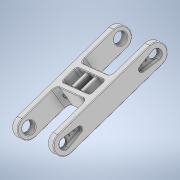
# Autodesk Inventor part: LegMiddle_Final_2
Saved by Autodesk Inventor 2020.3 (Build 243373000, 373)
## iProperties
Created: 2021-02-18
Part Number: LegMiddle_Final_2
Material: Generic
Document SubType Name: Modeling
Designer: sanyi
Density: 1 g/cm^3
Appearance: Default
Author: sanyi
Autodesk Inventor part; units mm, degrees
note: some values were not read from the file. Chosen so that the rebuilt part matches the saved one: direction of "Hole7"; direction of "Hole6".
ref_plane "YZ Plane" through (0, 0, 0) normal (1, 0, 0) x (0, 1, 0)
ref_plane "XZ Plane" through (0, 0, 0) normal (0, 1, 0) x (-1, 0, 0)
ref_plane "XY Plane" through (0, 0, 0) normal (0, 0, 1) x (1, 0, 0)
sketch "Sketch1" plane through (0, 0, 0) normal (0, 1, 0) x (-1, 0, 0)
  line L0 (0, 0) -> (0, 15.1754) construction
  line L1 (0, 0) -> (0, -18.4224) construction
  line L2 (0, 0) -> (12.9194, 0) construction
  line L3 (45, 17) -> (45, 23)
  line L4 (10, 17) -> (45, 17)
  line L5 (10, -17) -> (45, -17)
  line L6 (45, -17) -> (45, -23)
  line L7 (0, 0) -> (-12.9194, 0) construction
  line L8 (-45, 17) -> (-45, 23)
  line L9 (-10, 17) -> (-45, 17)
  line L10 (-10, -17) -> (-45, -17)
  line L11 (-45, -17) -> (-45, -23)
  line L12 (10, -17) -> (10, 17)
  line L13 (-10, -17) -> (-10, 17)
  line L14 (63, 0) -> (-63, 0) projected
  line L15 (-45, 23) -> (45, 23)
  line L16 (45, -23) -> (-45, -23)
  line L17 (-45, 34.0051) -> (-45, -29.7103) construction
  line L18 (45, 30.9627) -> (45, -32.2261) construction
  line L19 (0, -45.4724) -> (0, 47.2514) projected
  line L20 (45, 20) -> (-45, 20) construction
  dimension "d2" = 6
  dimension "d8" = 34
  dimension "d11" = 20
  dimension "d30" = 35
  dimension "d31" = 35
  constraints: 38 end point, 11 perpendicular, 6 point on line, 2 vertical, 6 other
  measures "d2" distance of L3.start L3.end
  measures "d8" distance of L4.start L5.start
  measures "d11" distance between parallel lines of L13 L12
  measures "d30" distance between parallel lines of L17 L13
  measures "d31" distance between parallel lines of L18 L12
extrude "Extrusion1" add sketch "Sketch1" along normal blind 15
sketch "Sketch2" plane through (0, 15, 0) normal (0, 1, 0) x (1, 0, 0)
  line L0 (-63, 0) -> (63, 0) projected
  line L1 (0, 32.2) -> (0, -32.2) projected
  line L2 (-6, -3) -> (6, -3)
  line L3 (6, -3) -> (6, 3)
  line L4 (6, 3) -> (-6, 3)
  line L5 (-6, 3) -> (-6, -3)
  line L6 (-6, -16) -> (6, -16)
  line L7 (6, -16) -> (6, -7)
  line L8 (6, -7) -> (-6, -7)
  line L9 (-6, -7) -> (-6, -16)
  line L10 (-6, 16) -> (6, 16)
  line L11 (6, 16) -> (6, 7)
  line L12 (6, 7) -> (-6, 7)
  line L13 (-6, 7) -> (-6, 16)
  line L14 (-6, -7) -> (-6, -3)
  line L15 (6, -7) -> (6, -3)
  line L16 (6, 3) -> (6, 7)
  line L17 (-6, 3) -> (-6, 7)
  line L18 (-10, -17) -> (-45, -17) projected
  point P0 (0, 0)
  dimension "d14" = 3
  dimension "d15" = 6
  dimension "d16" = 4
  dimension "d72" = 1
  constraints: 32 end point, 4 symmetric about line, 3 perpendicular, 2 collinear, 2 parallel, 1 horizontal, 1 vertical, 2 other
  measures "d14" distance between parallel lines of L4 L0
  measures "d15" distance between parallel lines of L3 L1
  measures "d16" distance between parallel lines of L2 L8
  measures "d72" distance between parallel lines of L18 L6
extrude "Extrusion2" cut sketch "Sketch2" against normal up to surface (15 mm away) contours L5 L4 L1 L0 | L0 L1 L2 L5 | L1 L4 L3 L0 | L0 L3 L2 L1 | L13 L10 L1 L12 | L8 L1 L6 L9 | L1 L10 L11 L12 | L8 L7 L6 L1
full round fillet "Fillet1" first side at (3.3333, 15, -21) centre faces at (-45, 5, -21) second side at (3.3333, 0, -21)
full round fillet "Fillet2" first side at (3.3333, 15, 21) centre faces at (45, 5, -19) second side at (3.3333, 0, 21)
full round fillet "Fillet3" first side at (3.3333, 15, 21) centre faces at (45, 5, 21) second side at (3.3333, 0, 21)
full round fillet "Fillet4" first side at (0.8334, 15, 21) centre faces at (-45, 5, 19) second side at (0.8334, 0, 21)
sketch "Sketch5" plane through (-37.5, 7.5, -23) normal (0, 0, -1) x (-1, 0, 0)
  arc A0 (0, -7.5) -> (0, 7.5) centre (0, 0) ccw projected
  arc A1 (-75, 7.5) -> (-75, -7.5) centre (-75, 0) ccw projected
  line L0 (-75, 0) -> (0, 0) construction
  circle A2 centre (0, 0) radius 3.6
  arc A3 (-12.3676, 1.8305) -> (-12.3676, -1.8305) centre (-12.1, 0) ccw
  line L1 (-0.5207, 3.5621) -> (-12.3676, 1.8305)
  line L2 (-12.3676, -1.8305) -> (-0.5207, -3.5621)
  circle A4 centre (-75, 0) radius 3.6
  arc A5 (-62.6324, -1.8305) -> (-62.6324, 1.8305) centre (-62.9, 0) ccw
  line L3 (-74.4793, 3.5621) -> (-62.6324, 1.8305)
  line L4 (-74.4793, -3.5621) -> (-62.6324, -1.8305)
  line L5 (-37.5, -7.5) -> (-37.5, 7.5)
  line L6 (-43.5, 7.5) -> (-31.5, 7.5) projected
  dimension "d53" = 3.7
  dimension "d54" = 12.1
  dimension "d76" = 12.1
  dimension "d89" = 7.2
  constraints: 12 end point, 8 point on circle, 8 tangent, 4 centre point, 2 coincident, 2 equal radius, 2 point on line, 1 horizontal, 1 midpoint
  measures "d53" diameter of A5
  measures "d54" distance of A5.centre L0.start
  measures "d76" distance of L0.end A3.centre
  measures "d89" diameter of A4
extrude "Extrusion4" cut sketch "Sketch5" against normal up to surface (6 mm away) contours A2 | A4
extrude "Extrusion5" cut sketch "Sketch5" against normal blind 3.5 contours A2 L2 A3 L1 | A4 L3 A5 L4
sketch "Sketch14" plane through (-37.5, 7.5, -19.5) normal (0, 0, -1) x (-1, 0, 0)
  arc A0 (-62.6324, -1.8305) -> (-62.6324, 1.8305) centre (-62.9, 0) ccw projected
  arc A1 (-12.3676, 1.8305) -> (-12.3676, -1.8305) centre (-12.1, 0) ccw projected
  line L0 (-62.9, 0) -> (-64.9, 0)
  line L1 (-12.1, 0) -> (-10.1, 0)
  line L2 (0, 7.5) -> (-75, 7.5) projected
  line L3 (0, -7.5) -> (-75, -7.5) projected
  line L4 (-37.5, 7.5) -> (-37.5, -7.5) construction
  line L5 (-75, 7.5) -> (-75, -7.5) construction
  line L6 (0, 7.5) -> (0, -7.5) construction
  line L7 (-75, 0) -> (0, 0) construction
  line L8 (-64.9, 0) -> (-66.9, 0)
  line L9 (-66.9, 0) -> (-68.9, 0)
  line L10 (-10.1, 0) -> (-8.1, 0)
  line L11 (-8.1, 0) -> (-6.1, 0)
  point P0 (-37.5, -7.5)
  point P1 (-12.1, 0)
  dimension "d121" = 2
  dimension "d122" = 2
  dimension "d123" = 2
  constraints: 20 end point, 8 coincident, 4 midpoint, 3 point on line, 3 symmetric about line, 2 vertical, 1 other
  measures "d121" distance of L0.start L0.end
  measures "d122" distance of L8.start L8.end
  measures "d123" distance of L8.end L9.end
hole "Hole7" at (27.4, 7.5, -19.5) at (31.4, 7.5, -19.5) at (-27.4, 7.5, -19.5) at (-31.4, 7.5, -19.5) direction (0, 0, 1) diameter 1 depth 2.5
extrude "Extrusion6" cut sketch "Sketch2" against normal blind 1 contours L17 L12 L1 L4 | L2 L1 L8 L14 | L1 L12 L16 L4 | L2 L15 L8 L1
sketch "Sketch6" plane through (0, 0, 0) normal (0, -1, 0) x (1, 0, 0)
  line L0 (6, 3) -> (6, 7) projected
  line L1 (6, 7) -> (-6, 7) projected
  line L2 (-6, 3) -> (6, 3) projected
  line L3 (-6, 7) -> (-6, 3) projected
  line L4 (6, -3) -> (-6, -3) projected
  line L5 (-6, -7) -> (6, -7) projected
  line L6 (-6, -3) -> (-6, -7) projected
  line L7 (6, -7) -> (6, -3) projected
  point P0 (0, 0)
extrude "Extrusion7" cut sketch "Sketch6" against normal blind 1
sketch "Sketch12" plane through (10, 0, 17) normal (1, 0, 0) x (0, 0, -1)
  line L0 (0, 0) -> (0, 15) projected
  line L1 (0, 7.5) -> (3, 7.5) construction
  point P0 (17, 0)
  dimension "d97" = 3
  constraints: 2 end point, 1 coincident, 1 horizontal, 1 midpoint
  measures "d97" distance of L1.start L1.end
hole "Hole5" at (10, 7.5, 14) direction (-1, 0, 0) diameter 3 end through all
fillet "Fillet13" radius 3.5 4 edges at (10, 7.5, 17) (-10, 7.5, 17) (-10, 7.5, -17) (10, 7.5, -17)
fillet "Fillet11" radius 2 4 edges at (-6, 7.5, -16) (6, 7.5, -16) (6, 7.5, 16) (-6, 7.5, 16)
fillet "Fillet9" radius 0.5 24 edges at (-6, 1, -5) (0, 1, -7) (0, 1, -3) (-6, 7.5, 3) (-6, 7.5, -7) (-6, 7.5, -3) (0, 14, -7) (0, 14, -3) (0, 1, 3) (0, 1, 7) (6, 1, -5) (6, 1, 5) (6, 7.5, -7) (6, 7.5, -3) (-6, 14, -5) (-6, 14, 5) (-6, 7.5, 7) (0, 14, 7) (0, 14, 3) (6, 14, 5) (6, 7.5, 3) (6, 7.5, 7) (-6, 1, 5) (6, 14, -5)
fillet "Fillet15" radius 0.5 16 edges at (5.4142, 15, 15.4142) (-5.4142, 15, 15.4142) (0, 15, 16) (-6, 15, 0) (5.4142, 15, -15.4142) (-5.4142, 15, -15.4142) (0, 15, -16) (6, 15, 0) (5.4142, 0, -15.4142) (-5.4142, 0, -15.4142) (0, 0, -16) (-6, 0, 0) (5.4142, 0, 15.4142) (-5.4142, 0, 15.4142) (0, 0, 16) (6, 0, 0)
fillet "Fillet12" radius 0.2 8 edges at (10, 8.366, 12.7753) (10, 6.634, 12.7753) (6, 8.5607, 12.9393) (6, 6.4393, 12.9393) (-6, 8.5607, 12.9393) (-6, 6.4393, 12.9393) (-10, 6.634, 12.7753) (-10, 8.366, 12.7753)
sketch "Sketch13" plane through (37.5, 7.5, 23) normal (0, 0, 1) x (1, 0, 0)
  arc A0 (-75, 7.5) -> (-75, -7.5) centre (-75, 0) ccw projected
  arc A1 (0, -7.5) -> (0, 7.5) centre (0, 0) ccw projected
  point P0 (-37.5, -7.5)
  constraints: 2 coincident
hole "Hole6" at (-37.5, 7.5, 23) at (37.5, 7.5, 23) direction (0, 0, -1) diameter 8.7 depth 6
fillet "Fillet14" radius 0.5 40 edges at (-11.0251, 15, 15.9749) (-25.5, 15, 17) (-42.8033, 2.1967, 17) (-42.8033, 12.8033, 17) (-25.5, 0, 17) (-11.0251, 0, 15.9749) (-10, 0, 0) (-11.0251, 0, -15.9749) (-25.5, 0, -17) (-42.8033, 12.8033, -17) (-42.8033, 2.1967, -17) (-25.5, 15, -17) (-11.0251, 15, -15.9749) (-10, 15, 0) (-42.8033, 2.1967, -23) (-42.8033, 12.8033, -23) (0, 0, -23) (42.8033, 12.8033, -23) (42.8033, 2.1967, -23) (0, 15, -23) (11.0251, 15, -15.9749) (25.5001, 15, -17) (42.8033, 12.8033, -17) (42.8033, 2.1967, -17) (25.5001, 0, -17) (11.0251, 0, -15.9749) (10, 0, 0) (11.0251, 0, 15.9749) (25.5001, 0, 17) (42.8033, 12.8033, 17) (42.8033, 2.1967, 17) (25.5001, 15, 17) (11.0251, 15, 15.9749) (10, 15, 0) (42.8033, 2.1967, 23) (42.8033, 12.8033, 23) (0, 0, 23) (-42.8033, 2.1967, 23) (-42.8033, 12.8033, 23) (0, 15, 23)
fillet "Fillet16" radius 0.5 4 edges at (37.5, 11.85, 17) (-37.5, 11.85, 17) (-33.9, 7.5, -17) (41.1, 7.5, -17)
fillet "Fillet17" radius 0.3 9 edges at (41.1, 7.5, -23) (31.0559, 10.1963, -23) (23.55, 7.5, -23) (31.0559, 4.8037, -23) (-23.55, 7.5, -23) (-31.0559, 10.1963, -23) (-39.8543, 4.7765, -23) (-39.8543, 10.2235, -23) (-31.0559, 4.8037, -23)
body "Solid1"
